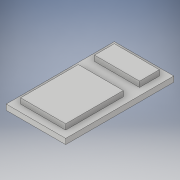
# Autodesk Inventor part: Colorimeter_Seal_Illumination
Saved by Autodesk Inventor 2019 (Build 230136000, 136)
## iProperties
Created: 2019-04-03
Part Number: Colorimeter_Seal_Illumination
Material: Generic
Document SubType Name: Modeling
Designer: Hansen
Density: 1 g/cm^3
Appearance: Default
Author: Hansen
Autodesk Inventor part; units mm, degrees
ref_plane "YZ Plane" through (0, 0, 0) normal (1, 0, 0) x (0, 1, 0)
ref_plane "XZ Plane" through (0, 0, 0) normal (0, 1, 0) x (-1, 0, 0)
ref_plane "XY Plane" through (0, 0, 0) normal (0, 0, 1) x (1, 0, 0)
sketch "Sketch1" plane through (0, 0, 0) normal (0, 1, 0) x (-1, 0, 0)
  line L0 (-8.25, 15) -> (8.25, 15)
  line L1 (8.25, 15) -> (8.25, -15)
  line L2 (8.25, -15) -> (-8.25, -15)
  line L3 (-8.25, -15) -> (-8.25, 15)
  line L4 (-8.25, 15) -> (8.25, -15) construction
  line L5 (8.25, 15) -> (-8.25, -15) construction
  point P0 (0, 0)
  dimension "d0" = 16.5
  dimension "d1" = 30
  constraints: 12 end point, 2 midpoint, 2 parallel, 1 horizontal, 1 perpendicular
  measures "d0" distance of L0.start L0.end
  measures "d1" distance of L0.end L1.end
extrude "Extrusion1" add sketch "Sketch1" along normal blind 1.5
sketch "Sketch2" plane through (0, 1.5, 0) normal (0, 1, 0) x (1, 0, 0)
  line L0 (6.25, -13) -> (-6.25, -13)
  line L1 (-6.25, -13) -> (-6.25, 3)
  line L2 (-6.25, 3) -> (6.25, 3)
  line L3 (6.25, 3) -> (6.25, -13)
  line L4 (6.25, -13) -> (-6.25, 3) construction
  line L5 (-6.25, -13) -> (6.25, 3) construction
  line L6 (6.25, 7.5) -> (-6.25, 7.5)
  line L7 (-6.25, 7.5) -> (-6.25, 13)
  line L8 (-6.25, 13) -> (6.25, 13)
  line L9 (6.25, 13) -> (6.25, 7.5)
  line L10 (6.25, 7.5) -> (-6.25, 13) construction
  line L11 (-6.25, 7.5) -> (6.25, 13) construction
  line L12 (-8.25, -15) -> (8.25, -15) projected
  line L13 (-8.25, 15) -> (-8.25, -15) projected
  line L14 (8.25, 15) -> (-8.25, 15) projected
  point P0 (0, 0)
  point P1 (0, -5)
  point P2 (0, 10.25)
  point P3 (0, -5)
  point P4 (0, 10.25)
  dimension "d4" = 2
  dimension "d5" = 2
  dimension "d6" = 16
  dimension "d7" = 2
  dimension "d8" = 5.5
  constraints: 24 end point, 6 midpoint, 4 parallel, 2 horizontal, 2 perpendicular, 2 vertical alignment, 1 point on line
  measures "d4" distance between parallel lines of L0 L12
  measures "d5" distance between parallel lines of L1 L13
  measures "d6" distance of L0.end L1.end
  measures "d7" distance between parallel lines of L14 L8
  measures "d8" distance between parallel lines of L8 L6
extrude "Extrusion2" add sketch "Sketch2" along normal blind 1.5
equation "\"d5\" = d4"
equation "\"d7\" = d4"
body "Solid1"
